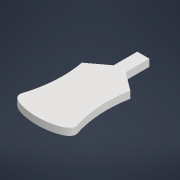
# Autodesk Inventor part: spatula
Saved by Autodesk Inventor 2021 (Build 250183000, 183)
## iProperties
Created: 2022-05-25
Part Number: spatula
Material: Generic
Document SubType Name: Modeling
Designer: techv
Density: 1 g/cm^3
Appearance: Default
Author: techv
Autodesk Inventor part; units mm, degrees
ref_plane "YZ Plane" through (0, 0, 0) normal (1, 0, 0) x (0, 1, 0)
ref_plane "XZ Plane" through (0, 0, 0) normal (0, 1, 0) x (-1, 0, 0)
ref_plane "XY Plane" through (0, 0, 0) normal (0, 0, 1) x (1, 0, 0)
sketch "Sketch1" plane through (0, 0, 0) normal (0, 1, 0) x (-1, 0, 0)
  line L0 (-24, 28) -> (24, 28) construction
  line L1 (24, 28) -> (24, -28) construction
  line L2 (24, -28) -> (-24, -28) construction
  line L3 (-24, -28) -> (-24, 28) construction
  line L4 (-24, 28) -> (24, -28) construction
  line L5 (24, 28) -> (-24, -28) construction
  line L6 (-27.5, -28) -> (27.5, -28) construction
  line L7 (27.5, -28) -> (27.5, 28) construction
  line L8 (27.5, 28) -> (-27.5, 28) construction
  line L9 (-27.5, 28) -> (-27.5, -28) construction
  line L10 (-27.5, -28) -> (27.5, 28) construction
  line L11 (27.5, -28) -> (-27.5, 28) construction
  line L12 (0, 28) -> (0, -28)
  line L13 (27.5, 28) -> (18.6445, 0) construction
  line L14 (18.6445, 0) -> (24, -28) construction
  spline S0 degree 2 poles (27.5, 28) (18.6445, 0) (24, -28) knots 1 1 1 2 2 2
  line L15 (27.5, 28) -> (30.2421, 36.6703) construction
  line L16 (30.2421, 36.6703) -> (12.6095, 40.7185) construction
  line L17 (12.6095, 40.7185) -> (0, 40.7185) construction
  spline S1 degree 3 poles (27.5, 28) (30.2421, 36.6703) (12.6095, 40.7185) (0, 40.7185) knots 1 1 1 1 2 2 2 2
  line L18 (24, -28) -> (6, -41.5)
  line L19 (6, -41.5) -> (6, -64.8839)
  line L20 (-27.5, 28) -> (-18.6445, 0) construction
  line L21 (-18.6445, 0) -> (-24, -28) construction
  spline S2 degree 2 poles (-27.5, 28) (-18.6445, 0) (-24, -28) knots 1 1 1 2 2 2
  line L22 (-27.5, 28) -> (-30.2421, 36.6703) construction
  line L23 (-30.2421, 36.6703) -> (-12.6095, 40.7185) construction
  line L24 (-12.6095, 40.7185) -> (0, 40.7185) construction
  spline S3 degree 3 poles (-27.5, 28) (-30.2421, 36.6703) (-12.6095, 40.7185) (0, 40.7185) knots 1 1 1 1 2 2 2 2
  line L25 (-24, -28) -> (-6, -41.5)
  line L26 (-6, -41.5) -> (-6, -64.8839)
  line L27 (6, -64.8839) -> (-6, -64.8839)
  point P0 (0, 0)
  dimension "d0" = 48
  dimension "d1" = 56
  dimension "d2" = 55
  dimension "d3" = 56
  dimension "d6" = 6
  dimension "d7" = 13.5
  constraints: 36 end point, 6 midpoint, 5 symmetric about line, 4 horizontal, 4 parallel, 2 perpendicular, 2 point on line, 1 vertical, 12 other
  measures "d0" distance of L1.end L2.end
  measures "d1" distance of L0.end L1.end
  measures "d2" distance of L8.end L7.end
  measures "d3" distance of L7.end L6.end
  measures "d6" distance between parallel lines of L12 L19
  measures "d7" vertical distance of L2.end L25.end
extrude "Extrusion1" add sketch "Sketch1" along normal blind 7
body "Solid1"
